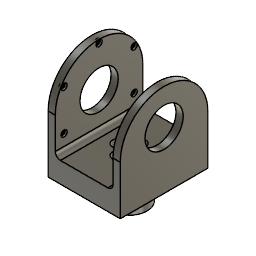
Joint 1 and 2 (Autodesk Fusion 360 archive; units mm, degrees)
design "Hinge"
Autodesk Fusion 360 part; units mm, degrees
sketch "Sketch1" plane through (0, 0, 0) normal (0, 0, 1) x (1, 0, 0)
  line L0 (0, 0) -> (70, 0)
  line L1 (70, 0) -> (70, 85)
  line L2 (70, 85) -> (0, 85)
  line L3 (0, 85) -> (0, 0)
  dimension "d1" = 70
  dimension "d2" = 85
  constraint horizontal L0
  constraint vertical L1
  constraint horizontal L2
  constraint vertical L3
  constraint coincident L0.start L3.end
  measures "d1" distance of L0.start L0.end
  measures "d2" distance of L0.start L2.end
extrude "Extrude1" add sketch "Sketch1" along normal blind 20
sketch "Sketch2" plane through (0, 0, 20) normal (0, 0, 1) x (-1, 0, 0)
  line L0 (0, -85) -> (0, 0)
  line L1 (0, 0) -> (-70, 0)
  line L2 (-70, 0) -> (-70, -85)
  line L3 (-70, -85) -> (0, -85)
  line L4 (-70, 0) -> (-63, 0)
  line L5 (-63, 0) -> (-63, -85)
  line L6 (-63, -85) -> (-70, -85)
  line L7 (-70, -85) -> (-70, 0)
  line L8 (0, 0) -> (-7, 0)
  line L9 (-7, 0) -> (-7, -85)
  line L10 (-7, -85) -> (0, -85)
  line L11 (0, -85) -> (0, 0)
  dimension "d5" = 7
  dimension "d6" = 7
  constraint horizontal L4
  constraint vertical L5
  constraint horizontal L6
  constraint vertical L7
  constraint coincident L1.end L2.start
  constraint horizontal L8
  constraint vertical L9
  constraint horizontal L10
  constraint vertical L11
  constraint coincident L0.end L1.start
  measures "d5" distance of L1.end L4.end
  measures "d6" distance of L0.end L8.end
extrude "Extrude2" add sketch "Sketch2" along normal blind 70 contours L1 L2 L3 L4 L5 L6 L7
extrude "Extrude3" add sketch "Sketch2" along normal blind 78 contours L0 L1 L3 L8 L9 L10 L11
sketch "Sketch3" plane through (0, 0, 0) normal (-1, 0, 0) x (0, -1, 0)
  line L0 (-85, 0) -> (0, 0)
  line L1 (0, 0) -> (0, 98)
  line L2 (0, 98) -> (-85, 98)
  line L3 (-85, 98) -> (-85, 0)
  circle A0 centre (-42.5, 55.5) radius 18.5
  dimension "d11" = 37
  dimension "d12" = 42.5
  dimension "d13" = 42.5
  measures "d11" diameter of A0
  measures "d12" distance of L2 A0.centre
  measures "d13" distance of L3 A0.centre
extrude "Extrude4" cut sketch "Sketch3" against normal blind 70 contours A0
fillet "Fillet1" radius 42.5 2 edges at (3.5, 0, 98) (3.5, 85, 98)
fillet "Fillet2" radius 42.5 2 edges at (66.5, 0, 90) (66.5, 85, 90)
fillet "Fillet3" radius 5 2 edges at (63, 42.5, 20) (7, 42.5, 20)
sketch "Sketch4" plane through (0, 0, 0) normal (-1, 0, 0) x (0, -1, 0)
  arc A0 (0, 55.5) -> (-85, 55.5) centre (-42.5, 55.5) ccw
  line L0 (-85, 55.5) -> (-85, 0)
  line L1 (-85, 0) -> (0, 0)
  line L2 (0, 0) -> (0, 55.5)
  circle A1 centre (-42.5, 55.5) radius 18.5
  circle A2 centre (-42.5, 55.5) radius 39.25
  circle A3 centre (-42.5, 94.75) radius 1.65
  circle A4 centre (-8.5085, 75.125) radius 1.65
  circle A5 centre (-76.4915, 75.125) radius 1.65
  circle A6 centre (-76.4915, 35.875) radius 1.65
  circle A7 centre (-8.5085, 35.875) radius 1.65
  line L3 (-42.5, 94.75) -> (-42.5, 55.5)
  line L4 (-42.5, 55.5) -> (-8.5085, 75.125)
  dimension "d22" = 78.5
  dimension "d23" = 3.3
  dimension "d24" = 3.3
  dimension "d25" = 3.3
  dimension "d26" = 3.3
  dimension "d27" = 3.3
  dimension "d65" = 60
  constraint concentric A0 A2
  constraint coincident A2 A3.centre
  constraint coincident A2 A5.centre
  constraint coincident A2 A6.centre
  constraint coincident A2 A7.centre
  constraint coincident A3.centre L3.start
  constraint coincident A0.centre A1.centre
  constraint vertical L3
  constraint coincident A2 A4.centre
  measures "d22" diameter of A2
  measures "d23" diameter of A3
  measures "d24" diameter of A4
  measures "d25" diameter of A5
  measures "d26" diameter of A6
  measures "d27" diameter of A7
  measures "d65" angle of L3 L4
extrude "Extrude5" cut sketch "Sketch4" against normal blind 7 contours A2 A4 L4 | A2 A4 L4 | A2 A3 L3 | A2 A3 L3 | A2 A4 | A2 A3 | A2 A5 | A2 A5 | A2 A7 | A2 A7 | A2 A6 | A2 A6
sketch "Sketch5" plane through (7, 0, 0) normal (1, 0, 0) x (0, 1, 0)
  circle A0 centre (76.4915, 35.875) radius 1.65
  circle A1 centre (76.4915, 75.125) radius 1.65
  circle A2 centre (8.5085, 35.875) radius 1.65
  circle A3 centre (42.5, 94.75) radius 1.65
  circle A4 centre (8.5085, 75.125) radius 1.65
  line L0 (0, 25) -> (85, 25)
  line L1 (85, 25) -> (85, 55.5)
  arc A5 (85, 55.5) -> (0, 55.5) centre (42.5, 55.5) ccw
  line L2 (0, 55.5) -> (0, 25)
  circle A6 centre (42.5, 55.5) radius 18.5
  circle A7 centre (42.5, 94.75) radius 3
  circle A8 centre (76.4915, 75.125) radius 3
  circle A9 centre (8.5085, 75.125) radius 3
  circle A10 centre (8.5085, 35.875) radius 3
  circle A11 centre (76.4915, 35.875) radius 3
  dimension "d30" = 6
  dimension "d31" = 6
  dimension "d32" = 6
  dimension "d33" = 6
  dimension "d34" = 6
  constraint concentric A3 A7
  constraint concentric A1 A8
  constraint concentric A4 A9
  constraint concentric A2 A10
  constraint concentric A0 A11
  measures "d30" diameter of A7
  measures "d31" diameter of A8
  measures "d32" diameter of A9
  measures "d33" diameter of A10
  measures "d34" diameter of A11
extrude "Extrude6" cut sketch "Sketch5" against normal blind 2 contours A7 | A8 | A9 | A10 | A11
sketch "Sketch6" plane through (0, 0, 0) normal (0, 0, -1) x (1, 0, 0)
  line L0 (0, 0) -> (0, -85)
  line L1 (0, -85) -> (70, -85)
  line L2 (70, -85) -> (70, 0)
  line L3 (70, 0) -> (0, 0)
  circle A0 centre (36, -42.5) radius 30.5
  point P0 (58, -42.5)
  point P1 (36, -42.5)
  dimension "d37" = 42.5
  dimension "d38" = 12
  dimension "d39" = 22
  dimension "d40" = 42.5
  dimension "d41" = 61
  constraint coincident P1 A0.centre
  measures "d37" distance of L3 P0
  measures "d38" distance of L2 P0
  measures "d39" distance of P0 P1
  measures "d40" distance of L3 P1
  measures "d41" diameter of A0
extrude "Extrude7" cut sketch "Sketch6" against normal blind 10 contours A0
sketch "Sketch7" plane through (0, 0, 10) normal (0, 0, -1) x (1, 0, 0)
  circle A0 centre (36, -42.5) radius 30.5
  circle A1 centre (36, -42.5) radius 17.5
  dimension "d44" = 35
  constraint concentric A0 A1
  measures "d44" diameter of A1
extrude "Extrude8" add sketch "Sketch7" along normal blind 33 contours A1
sketch "Sketch8" plane through (0, 0, -23) normal (0, 0, -1) x (1, 0, 0)
  circle A0 centre (36, -42.5) radius 17.5
  circle A1 centre (36, -32.5) radius 2.65
  circle A2 centre (36, -52.5) radius 2.65
  circle A3 centre (46, -42.5) radius 2.65
  circle A4 centre (26, -42.5) radius 2.65
  dimension "d47" = 5.3
  dimension "d48" = 10
  dimension "d49" = 5.3
  dimension "d50" = 10
  dimension "d51" = 5.3
  dimension "d52" = 10
  dimension "d53" = 5.3
  dimension "d54" = 10
  dimension "d55" = 10
  dimension "d56" = 10
  measures "d47" diameter of A1
  measures "d48" distance of A0.centre A1.centre
  measures "d49" diameter of A2
  measures "d50" distance of A0.centre A2.centre
  measures "d51" diameter of A3
  measures "d52" distance of A0.centre A3.centre
  measures "d53" diameter of A4
  measures "d54" distance of A0.centre A4.centre
  measures "d55" vertical distance of A2.centre A3.centre
  measures "d56" vertical distance of A2.centre A4.centre
extrude "Extrude9" cut sketch "Sketch8" against normal blind 48 contours A1 | A2 | A3 | A4
sketch "Sketch9" plane through (0, 0, 20) normal (0, 0, 1) x (-1, 0, 0)
  circle A0 centre (-36, -32.5) radius 2.65
  circle A1 centre (-26, -42.5) radius 2.65
  circle A2 centre (-46, -42.5) radius 2.65
  circle A3 centre (-36, -52.5) radius 2.65
  line L0 (-12, -85) -> (-12, 0)
  line L1 (-12, 0) -> (-58, 0)
  line L2 (-58, 0) -> (-58, -85)
  line L3 (-58, -85) -> (-12, -85)
  circle A4 centre (-36, -52.5) radius 6
  circle A5 centre (-26, -42.5) radius 6
  circle A6 centre (-46, -42.5) radius 6
  circle A7 centre (-36, -32.5) radius 6
  dimension "d59" = 12
  dimension "d60" = 12
  dimension "d61" = 12
  dimension "d62" = 12
  constraint concentric A3 A4
  constraint concentric A1 A5
  constraint concentric A2 A6
  constraint concentric A0 A7
  measures "d59" diameter of A4
  measures "d60" diameter of A5
  measures "d61" diameter of A6
  measures "d62" diameter of A7
extrude "Extrude10" cut sketch "Sketch9" against normal blind 12 contours A4 | A5 | A6 | A7

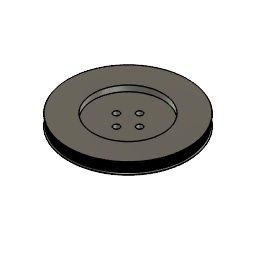
design "GT2-120"
Autodesk Fusion 360 part; units mm, degrees
sketch "Pulley Cylinder" plane through (0, 0, 0) normal (0, 0, 1) x (1, 0, 0) in component "Component"
  circle A0 centre (0, 0) radius 50.675582
extrude "Extrude1" add sketch "Pulley Cylinder" along normal blind 7 contours A0 picked at (-11.093693, -15.667951) in component "Component"
ref_plane "WorkPlane1" through (0, 0, 7) normal (0, 0, 1) x (1, 0, 0) in component "Component"
sketch "Sketch2" plane through (0, 0, 7) normal (0, 0, 1) x (1, 0, 0) in component "Component"
  circle A0 centre (0, 0) radius 51.675582
ref_plane "WorkPlane2" through (0, 0, 0) normal (0, 0, 1) x (1, 0, 0) in component "Component"
sketch "Sketch3" plane through (0, 0, 0) normal (0, 0, 1) x (1, 0, 0) in component "Component"
  circle A0 centre (0, 0) radius 51.675582
extrude "Extrude2" add sketch "Sketch2" along normal blind 1.5 contours A0 picked at (-10.126036, -19.823905) in component "Component"
extrude "Extrude3" add sketch "Sketch3" against normal blind 1.5 contours A0 picked at (-10.126036, -19.823905) in component "Component"
chamfer "Chamfer1" distance 1 angle 45 1 edges at (-48.178558, -18.686688, 0) in component "Component"
chamfer "Chamfer2" distance 1 angle 45 1 edges at (-48.178558, -18.686688, 7) in component "Component"
chamfer "Chamfer3" distance 0.2 angle 45 1 edges at (-48.178558, 18.686688, -1.5) in component "Component"
chamfer "Chamfer4" distance 0.2 angle 45 1 edges at (-48.178558, -18.686688, 8.5) in component "Component"
sketch "Bore" plane through (0, 0, 0) normal (0, 0, 1) x (1, 0, 0) in component "Component"
  circle A0 centre (0, 0) radius 1.5
  constraint coincident A0.centre origin
extrude "Extrude4" cut sketch "Bore" along normal blind 8.5 and the other way blind 1.5 contours A0 picked at (0.826239, -0.56332) in component "Component"
sketch "Tooth Profile" plane through (0, 0, 0) normal (0, 0, 1) x (1, 0, 0) in component "Component"
  circle A0 centre (0, 0) radius 50.675582 construction
  line L0 (-76.013373, 0) -> (76.013373, 0) construction
  line L1 (50.675582, -50.675582) -> (50.675582, 50.675582) construction
  line L2 (49.773989, 0.401771) -> (50.673989, 0.401771) construction
  line L3 (49.773989, -0.401771) -> (50.673989, -0.401771) construction
  arc A1 (50.097805, 0.401771) -> (50.097805, -0.401771) centre (50.48033, 0) ccw
  line L4 (49.925582, 0.4) -> (49.925582, -0.4) construction
  line L5 (50.097805, 0.401771) -> (50.097805, -0.401771) construction
  arc A2 (50.230073, -0.494298) -> (50.540254, -0.589246) centre (50.673989, 0.401771) ccw
  arc A3 (50.540254, 0.589247) -> (50.230083, 0.494303) centre (50.673989, -0.401771) ccw
  arc A4 (50.540254, 0.589247) -> (50.670177, 0.74009) centre (50.520193, 0.737899) ccw
  arc A5 (50.230083, 0.494303) -> (50.097805, 0.401771) centre (50.469126, 0.011768) ccw
  arc A6 (50.670177, -0.740089) -> (50.540254, -0.589246) centre (50.520193, -0.737899) ccw
  arc A7 (50.097805, -0.401771) -> (50.230073, -0.494298) centre (50.469115, -0.01178) ccw
  arc A8 (50.670177, -0.740089) -> (50.670177, 0.74009) centre (0, 0) ccw
  point P0 (50.48033, 0)
  point P1 (50.480582, 0)
  point P2 (50.480582, 0)
  dimension "d17" = 101.351164
  dimension "d18" = 0.803543
  dimension "d19" = 0.75
  dimension "d20" = 0.577777
  dimension "d21" = 1
  dimension "d22" = 1
  dimension "d23" = 0.15
  dimension "d24" = 0.15
  constraint coincident A0.centre A8.centre
  constraint midpoint A0.centre L0
  constraint horizontal L0
  constraint vertical L1
  constraint tangent A0 L1
  constraint horizontal L2
  constraint vertical L4
  constraint tangent A1 L4
  constraint tangent A3 A4
  constraint tangent A0 A4
  constraint tangent A1 A5
  constraint tangent A3 A5
  constraint tangent A2 A6
  constraint tangent A0 A6
  constraint tangent A1 A7
  constraint tangent A2 A7
  measures "d17" diameter of A0
  measures "d21" radius of A2
  measures "d22" radius of A3
  measures "d23" radius of A4
  measures "d24" radius of A6
extrude "Extrude5" cut sketch "Tooth Profile" along normal blind 7 contours A1 A2 A3 A4 A5 A6 A7 A8 picked at (50.425682, 0.013603) in component "Component"
pattern_circular "C-Pattern1" count 160 over 360 about axis through (0, 0, 1.75) along (0, 0, 1) of "Extrude5" in component "Component"
sketch "Sketch1" plane through (0, 0, 8.5) normal (0, 0, 1) x (-1, 0, 0)
  circle A0 centre (0, 0) radius 1.5
  circle A1 centre (0, 0) radius 51.475582
  circle A2 centre (0, 0) radius 30
  dimension "d29" = 60
  constraint coincident A0.centre A1.centre
  measures "d29" diameter of A2
extrude "Extrude6" cut sketch "Sketch1" against normal blind 5 contours A2 picked at (20.382724, -1.564944) in component "Component"
sketch "Sketch2 (2)" plane through (0, 0, 3.5) normal (0, 0, 1) x (-1, 0, 0)
  circle A0 centre (0, 0) radius 1.5
  circle A1 centre (0, 0) radius 30
  circle A2 centre (0, -10) radius 2.65
  circle A3 centre (10, 0) radius 2.65
  circle A4 centre (0, 10) radius 2.65
  circle A5 centre (-10, 0) radius 2.65
  dimension "d32" = 5.3
  dimension "d33" = 10
  dimension "d34" = 5.3
  dimension "d35" = 10
  dimension "d36" = 5.3
  dimension "d37" = 10
  dimension "d38" = 5.3
  dimension "d39" = 10
  measures "d32" diameter of A2
  measures "d33" distance of A0.centre A2.centre
  measures "d34" diameter of A3
  measures "d35" distance of A0.centre A3.centre
  measures "d36" diameter of A4
  measures "d37" distance of A0.centre A4.centre
  measures "d38" diameter of A5
  measures "d39" distance of A0.centre A5.centre
extrude "Extrude7" cut sketch "Sketch2 (2)" against normal blind 5 contours A2 | A3 | A4 | A5 picked at (0.676907, -9.00716) picked at (10.424592, 0.99284) picked at (0.921701, 9.488023) picked at (-9.581274, 0.690618) in component "Component"
delete_face "DeleteFace1" 1 faces at (1.498135, -0.074769, 1.833333) in component "Component"
sketch "Sketch3 (2)" plane through (0, 0, -1.5) normal (0, 0, -1) x (1, 0, 0)
  circle A0 centre (-10, 0) radius 2.65
  circle A1 centre (0, 10) radius 2.65
  circle A2 centre (0, -10) radius 2.65
  circle A3 centre (10, 0) radius 2.65
  circle A4 centre (0, 0) radius 51.475582
  circle A5 centre (0, 0) radius 4
  dimension "d42" = 8
  constraint coincident A4.centre A5.centre
  measures "d42" diameter of A5
extrude "Extrude8" add sketch "Sketch3 (2)" along normal blind 12 contours A5 picked at (-1.245636, 0.013218) in component "Component"
component "Component" placed x (1, 0, 0) y (0, 1, 0) z (0, 0, 1) at (0, 0, 0)
named bodies: "GT2 Pulley"

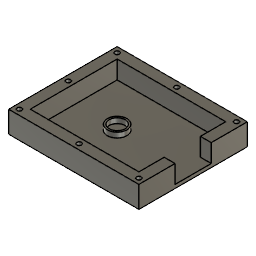
design "Box bottom"
Autodesk Fusion 360 part; units mm, degrees
sketch "Sketch1" plane through (0, 0, 0) normal (0, 0, 1) x (1, 0, 0)
  line L0 (0, 0) -> (180, 0)
  line L1 (180, 0) -> (180, 150)
  line L2 (180, 150) -> (0, 150)
  line L3 (0, 150) -> (0, 0)
  dimension "d1" = 180
  dimension "d2" = 150
  constraint horizontal L0
  constraint vertical L1
  constraint horizontal L2
  constraint vertical L3
  constraint coincident L0.start L3.end
  measures "d1" distance of L0.start L0.end
  measures "d2" distance of L0.start L2.end
extrude "Extrude1" add sketch "Sketch1" along normal blind 5
sketch "Sketch2" plane through (0, 0, 5) normal (0, 0, 1) x (-1, 0, 0)
  line L0 (0, -150) -> (0, 0)
  line L1 (0, 0) -> (-180, 0)
  line L2 (-180, 0) -> (-180, -150)
  line L3 (-180, -150) -> (0, -150)
  circle A0 centre (-75, -75) radius 11
  circle A1 centre (-75, -75) radius 13.5
  dimension "d5" = 22
  dimension "d6" = 75
  dimension "d7" = 75
  dimension "d8" = 27
  constraint concentric A0 A1
  measures "d5" diameter of A0
  measures "d6" distance of L3 A0.centre
  measures "d7" distance of L0 A0.centre
  measures "d8" diameter of A1
extrude "Extrude2" add sketch "Sketch2" along normal blind 7 contours A1
sketch "Sketch3" plane through (0, 0, 5) normal (0, 0, 1) x (-1, 0, 0)
  line L0 (0, -150) -> (0, 0)
  line L1 (0, 0) -> (-180, 0)
  line L2 (-180, 0) -> (-180, -150)
  line L3 (-180, -150) -> (0, -150)
  circle A0 centre (-75, -75) radius 13.5
  line L4 (-15, -15) -> (-165, -15)
  line L5 (-165, -135) -> (-15, -135)
  line L6 (-15, -135) -> (-15, -15)
  line L7 (-165, -50) -> (-180, -50)
  line L8 (-165, -100) -> (-180, -100)
  line L9 (-165, -135) -> (-165, -100)
  line L10 (-165, -15) -> (-165, -50)
  dimension "d11" = 150
  dimension "d12" = 120
  dimension "d13" = 15
  dimension "d14" = 15
  dimension "d17" = 25
  dimension "d18" = 25
  constraint horizontal L4
  constraint horizontal L5
  constraint vertical L6
  constraint coincident L2 L7.end
  constraint perpendicular L2 L7
  constraint coincident L2 L8.end
  constraint perpendicular L2 L8
  constraint perpendicular L8 L9
  constraint perpendicular L7 L10
  measures "d11" distance of L4.start L4.end
  measures "d12" distance of L4.start L5.end
  measures "d13" distance of L0 L6
  measures "d14" distance of L1 L4
  measures "d17" distance of A0.centre L7
  measures "d18" distance of A0.centre L8
extrude "Extrude4" add sketch "Sketch3" along normal blind 25 contours L0 L1 L2 L3 L4 L5 L6 L7 L8 L9 L10
sketch "Sketch4" plane through (0, 0, 30) normal (0, 0, 1) x (-1, 0, 0)
  line L0 (-165, -135) -> (-165, -100)
  line L1 (-165, -100) -> (-180, -100)
  line L2 (-180, -100) -> (-180, -150)
  line L3 (-180, -150) -> (0, -150)
  line L4 (0, -150) -> (0, 0)
  line L5 (0, 0) -> (-180, 0)
  line L6 (-180, 0) -> (-180, -50)
  line L7 (-180, -50) -> (-165, -50)
  line L8 (-165, -50) -> (-165, -15)
  line L9 (-165, -15) -> (-15, -15)
  line L10 (-15, -15) -> (-15, -135)
  line L11 (-15, -135) -> (-165, -135)
  circle A0 centre (-7.5, -142.5) radius 3.2
  circle A1 centre (-7.5, -75) radius 3.2
  circle A2 centre (-7.5, -7.5) radius 3.2
  circle A3 centre (-172.5, -7.5) radius 3.2
  circle A4 centre (-172.5, -142.5) radius 3.2
  circle A5 centre (-90, -142.5) radius 3.2
  circle A6 centre (-90, -7.5) radius 3.2
  dimension "d21" = 6.4
  dimension "d22" = 7.5
  dimension "d23" = 7.5
  dimension "d24" = 6.4
  dimension "d25" = 7.5
  dimension "d26" = 6.4
  dimension "d27" = 7.5
  dimension "d28" = 7.5
  dimension "d29" = 6.4
  dimension "d30" = 7.5
  dimension "d31" = 7.5
  dimension "d32" = 6.4
  dimension "d33" = 7.5
  dimension "d34" = 7.5
  dimension "d35" = 6.4
  dimension "d36" = 7.5
  dimension "d37" = 90
  dimension "d38" = 6.4
  dimension "d39" = 7.5
  dimension "d40" = 90
  measures "d21" diameter of A0
  measures "d22" distance of L3 A0.centre
  measures "d23" distance of L4 A0.centre
  measures "d24" diameter of A1
  measures "d25" distance of L4 A1.centre
  measures "d26" diameter of A2
  measures "d27" distance of L4 A2.centre
  measures "d28" distance of L5 A2.centre
  measures "d29" diameter of A3
  measures "d30" distance of L6 A3.centre
  measures "d31" distance of L5 A3.centre
  measures "d32" diameter of A4
  measures "d33" distance of L2 A4.centre
  measures "d34" distance of L3 A4.centre
  measures "d35" diameter of A5
  measures "d36" distance of L3 A5.centre
  measures "d37" distance of L2 A5.centre
  measures "d38" diameter of A6
  measures "d39" distance of L5 A6.centre
  measures "d40" distance of L6 A6.centre
extrude "Extrude5" cut sketch "Sketch4" against normal blind 10.5 contours A0 | A1 | A2 | A3 | A4 | A5 | A6

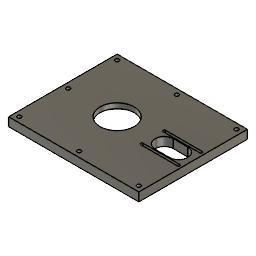
design "Box top"
Autodesk Fusion 360 part; units mm, degrees
sketch "Sketch1" plane through (0, 0, 0) normal (0, 0, 1) x (1, 0, 0)
  line L0 (0, 0) -> (180, 0)
  line L1 (180, 0) -> (180, 150)
  line L2 (180, 150) -> (0, 150)
  line L3 (0, 150) -> (0, 0)
  dimension "d1" = 180
  dimension "d2" = 150
  constraint horizontal L0
  constraint vertical L1
  constraint horizontal L2
  constraint vertical L3
  constraint coincident L0.start L3.end
  measures "d1" distance of L0.start L0.end
  measures "d2" distance of L0.start L2.end
extrude "Extrude1" add sketch "Sketch1" along normal blind 12
sketch "Sketch3" plane through (0, 0, 0) normal (0, 0, -1) x (1, 0, 0)
  line L0 (0, 0) -> (0, -150)
  line L1 (0, -150) -> (180, -150)
  line L2 (180, -150) -> (180, 0)
  line L3 (180, 0) -> (0, 0)
  circle A0 centre (75, -75) radius 30
  dimension "d8" = 60
  measures "d8" diameter of A0
extrude "Extrude3" cut sketch "Sketch3" against normal blind 5 contours A0
sketch "Sketch5" plane through (0, 0, 5) normal (0, 0, -1) x (1, 0, 0)
  circle A0 centre (75, -75) radius 30
  circle A1 centre (75, -75) radius 23.5
  dimension "d14" = 47
  constraint concentric A0 A1
  measures "d14" diameter of A1
extrude "Extrude5" cut sketch "Sketch5" against normal blind 12 contours A1
sketch "Sketch6" plane through (0, 0, 0) normal (0, 0, -1) x (1, 0, 0)
  circle A0 centre (75, -75) radius 30
  line L0 (0, 0) -> (0, -150)
  line L1 (0, -150) -> (180, -150)
  line L2 (180, -150) -> (180, 0)
  line L3 (180, 0) -> (0, 0)
  line L4 (140, -87.5) -> (160, -87.5)
  line L5 (160, -62.5) -> (140, -62.5)
  arc A1 (140, -62.5) -> (140, -87.5) centre (140, -75) ccw
  arc A2 (160, -87.5) -> (160, -62.5) centre (160, -75) ccw
  line L6 (175.5, -61.15) -> (124.5, -61.15)
  line L7 (124.5, -57.85) -> (175.5, -57.85)
  arc A3 (124.5, -57.85) -> (124.5, -61.15) centre (124.5, -59.5) ccw
  arc A4 (175.5, -61.15) -> (175.5, -57.85) centre (175.5, -59.5) ccw
  line L8 (175.5, -88.85) -> (124.5, -88.85)
  line L9 (124.5, -92.15) -> (175.5, -92.15)
  arc A5 (124.5, -88.85) -> (124.5, -92.15) centre (124.5, -90.5) ccw
  arc A6 (175.5, -92.15) -> (175.5, -88.85) centre (175.5, -90.5) ccw
  dimension "d17" = 25
  dimension "d18" = 20
  dimension "d19" = 20
  dimension "d20" = 51
  dimension "d22" = 15.5
  dimension "d23" = 3.3
  dimension "d24" = 51
  dimension "d25" = 3.3
  dimension "d29" = 15.5
  dimension "d30" = 15.5
  dimension "d31" = 75
  constraint horizontal L4
  constraint parallel L3 L5
  constraint tangent L5 A1
  constraint tangent L4 A1
  constraint tangent L5 A2
  constraint tangent L4 A2
  constraint horizontal L6
  constraint perpendicular L2 L7
  constraint tangent L7 A3
  constraint tangent L6 A3
  constraint tangent L7 A4
  constraint tangent L6 A4
  constraint parallel L6 L8
  constraint parallel L8 L9
  constraint tangent L8 A5
  constraint tangent L9 A5
  constraint tangent L8 A6
  constraint tangent L9 A6
  measures "d17" distance of L4 L5
  measures "d18" distance of A1.centre A2.centre
  measures "d19" distance of L2 A2.centre
  measures "d20" distance of L6.start L6.end
  measures "d22" horizontal distance of A1.centre L6.end
  measures "d23" distance of L6 L7
  measures "d24" distance of L8.start L8.end
  measures "d25" distance of L8 L9
  measures "d29" vertical distance of A1.centre A3.centre
  measures "d30" vertical distance of A1.centre A5.centre
  measures "d31" distance of L3 A2.centre
extrude "Extrude6" cut sketch "Sketch6" against normal blind 12 contours L4 L5 A1 A2 | L6 L7 A3 A4 | L8 L9 A5 A6
sketch "Sketch7" plane through (0, 0, 12) normal (0, 0, 1) x (-1, 0, 0)
  line L0 (-124.5, -61.15) -> (-175.5, -61.15)
  arc A0 (-175.5, -57.85) -> (-175.5, -61.15) centre (-175.5, -59.5) ccw
  line L1 (-175.5, -57.85) -> (-124.5, -57.85)
  arc A1 (-124.5, -61.15) -> (-124.5, -57.85) centre (-124.5, -59.5) ccw
  line L2 (-160, -62.5) -> (-140, -62.5)
  arc A2 (-140, -87.5) -> (-140, -62.5) centre (-140, -75) ccw
  line L3 (-140, -87.5) -> (-160, -87.5)
  arc A3 (-160, -62.5) -> (-160, -87.5) centre (-160, -75) ccw
  line L4 (-175.5, -88.85) -> (-124.5, -88.85)
  arc A4 (-124.5, -92.15) -> (-124.5, -88.85) centre (-124.5, -90.5) ccw
  line L5 (-124.5, -92.15) -> (-175.5, -92.15)
  arc A5 (-175.5, -88.85) -> (-175.5, -92.15) centre (-175.5, -90.5) ccw
  circle A6 centre (-75, -75) radius 23.5
  line L6 (0, -150) -> (0, 0)
  line L7 (0, 0) -> (-180, 0)
  line L8 (-180, 0) -> (-180, -150)
  line L9 (-180, -150) -> (0, -150)
  circle A7 centre (-7.5, -7.5) radius 2.65
  circle A8 centre (-7.5, -142.5) radius 2.65
  circle A9 centre (-172.5, -142.5) radius 2.65
  circle A10 centre (-172.5, -7.5) radius 2.65
  circle A11 centre (-90, -7.5) radius 2.65
  circle A12 centre (-90, -142.5) radius 2.65
  circle A13 centre (-7.5, -75) radius 2.65
  dimension "d32" = 5.3
  dimension "d33" = 7.5
  dimension "d34" = 7.5
  dimension "d35" = 5.3
  dimension "d36" = 7.5
  dimension "d37" = 7.5
  dimension "d38" = 5.3
  dimension "d39" = 7.5
  dimension "d40" = 7.5
  dimension "d41" = 5.3
  dimension "d42" = 7.5
  dimension "d43" = 7.5
  dimension "d44" = 5.3
  dimension "d45" = 90
  dimension "d46" = 7.5
  dimension "d47" = 5.3
  dimension "d48" = 7.5
  dimension "d49" = 90
  dimension "d50" = 5.3
  dimension "d51" = 7.5
  measures "d32" diameter of A7
  measures "d33" distance of L6 A7.centre
  measures "d34" distance of L7 A7.centre
  measures "d35" diameter of A8
  measures "d36" distance of L9 A8.centre
  measures "d37" distance of L6 A8.centre
  measures "d38" diameter of A9
  measures "d39" distance of L9 A9.centre
  measures "d40" distance of L8 A9.centre
  measures "d41" diameter of A10
  measures "d42" distance of L8 A10.centre
  measures "d43" distance of L7 A10.centre
  measures "d44" diameter of A11
  measures "d45" distance of L6 A11.centre
  measures "d46" distance of L7 A11.centre
  measures "d47" diameter of A12
  measures "d48" distance of L9 A12.centre
  measures "d49" distance of L8 A12.centre
  measures "d50" diameter of A13
  measures "d51" distance of L6 A13.centre
extrude "Extrude7" cut sketch "Sketch7" against normal blind 12 contours A7 | A8 | A9 | A10 | A11 | A12 | A13

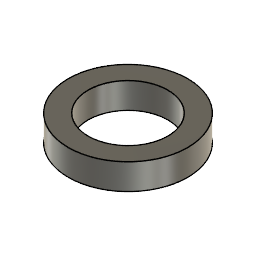
design "Thrust bearing 40x60x13"
Autodesk Fusion 360 part; units mm, degrees
sketch "Sketch1" plane through (0, 0, 0) normal (0, 0, 1) x (1, 0, 0)
  circle A0 centre (0, 0) radius 30
  circle A1 centre (0, 0) radius 20
  dimension "d1" = 60
  dimension "d2" = 40
  constraint coincident A0.centre A1.centre
  measures "d1" diameter of A0
  measures "d2" diameter of A1
extrude "Extrude1" add sketch "Sketch1" along normal blind 13

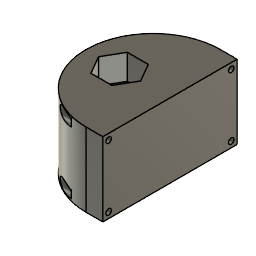
design "Coupling shaft"
Autodesk Fusion 360 part; units mm, degrees
sketch "Sketch1" plane through (0, 0, 0) normal (1, 0, 0) x (0, 1, 0)
  line L0 (0, 0) -> (-80, 0)
  line L1 (-80, 0) -> (-80, 44)
  line L2 (-80, 44) -> (0, 44)
  line L3 (0, 44) -> (0, 0)
  dimension "d1" = 80
  dimension "d2" = 44
  constraint horizontal L0
  constraint vertical L1
  constraint horizontal L2
  constraint vertical L3
  constraint coincident L0.start L3.end
  measures "d1" distance of L0.start L0.end
  measures "d2" distance of L0.start L2.end
extrude "Extrude1" add sketch "Sketch1" along normal blind 50
sketch "Sketch3" plane through (0, 0, 0) normal (-1, 0, 0) x (0, -1, 0)
  line L0 (80, 44) -> (0, 44)
  line L1 (0, 44) -> (0, 0)
  line L2 (0, 0) -> (80, 0)
  line L3 (80, 0) -> (80, 44)
  circle A0 centre (3.5, 40.5) radius 1.65
  circle A1 centre (3.5, 3.5) radius 1.65
  circle A2 centre (76.5, 40.5) radius 1.65
  circle A3 centre (76.5, 3.5) radius 1.65
  dimension "d17" = 3.3
  dimension "d18" = 3.5
  dimension "d19" = 3.5
  dimension "d20" = 3.3
  dimension "d21" = 3.5
  dimension "d22" = 3.3
  dimension "d23" = 3.5
  dimension "d24" = 3.3
  measures "d17" diameter of A0
  measures "d18" distance of L0 A0.centre
  measures "d19" distance of L1 A0.centre
  measures "d20" diameter of A1
  measures "d21" distance of L2 A1.centre
  measures "d22" diameter of A2
  measures "d23" distance of L3 A2.centre
  measures "d24" diameter of A3
extrude "Extrude3" cut sketch "Sketch3" against normal blind 50 contours A0 | A1 | A2 | A3
sketch "Sketch6" plane through (0, 0, 0) normal (-1, 0, 0) x (0, -1, 0)
  circle A0 centre (76.5, 40.5) radius 1.65
  circle A1 centre (76.5, 3.5) radius 1.65
  circle A2 centre (3.5, 40.5) radius 1.65
  circle A3 centre (3.5, 3.5) radius 1.65
  line L0 (80, 44) -> (0, 44)
  line L1 (0, 44) -> (0, 0)
  line L2 (0, 0) -> (80, 0)
  line L3 (80, 0) -> (80, 44)
  circle A4 centre (3.5, 40.5) radius 3
  circle A5 centre (3.5, 3.5) radius 3
  circle A6 centre (76.5, 40.5) radius 3
  circle A7 centre (76.5, 3.5) radius 3
  dimension "d46" = 6
  dimension "d47" = 6
  dimension "d48" = 6
  dimension "d49" = 6
  constraint concentric A2 A4
  constraint concentric A3 A5
  constraint concentric A0 A6
  constraint concentric A1 A7
  measures "d46" diameter of A4
  measures "d47" diameter of A5
  measures "d48" diameter of A6
  measures "d49" diameter of A7
extrude "Extrude7" cut sketch "Sketch6" against normal blind 30 contours A4 | A5 | A6 | A7
sketch "Sketch7" plane through (0, 0, 0) normal (0, 0, -1) x (1, 0, 0)
  line L0 (0, 80) -> (0, 0)
  line L1 (0, 0) -> (50, 0)
  line L2 (50, 0) -> (50, 80)
  line L3 (50, 80) -> (0, 80)
  circle A0 centre (20, 40) radius 16.5
  dimension "d52" = 33
  dimension "d53" = 20
  measures "d52" diameter of A0
  measures "d53" distance of L0 A0.centre
extrude "Extrude8" add sketch "Sketch7" along normal blind 3 contours A0
sketch "Sketch8" plane through (0, 0, -3) normal (0, 0, -1) x (1, 0, 0)
  circle A0 centre (20, 40) radius 16.5
  circle A1 centre (20, 40) radius 14.5
  dimension "d56" = 29
  constraint concentric A0 A1
  measures "d56" diameter of A1
extrude "Extrude9" add sketch "Sketch8" along normal blind 2 contours A1
fillet "Fillet1" radius 14 1 edges at (4.6166, -34.0333, -3)
sketch "Sketch9" plane through (0, 0, -5) normal (0, 0, -1) x (1, 0, 0)
  circle A0 centre (20, 40) radius 14.5
  circle A1 centre (20, 40) radius 12.5
  dimension "d61" = 25
  constraint concentric A0 A1
  measures "d61" diameter of A1
extrude "Extrude10" add sketch "Sketch9" along normal blind 7 contours A1
sketch "Sketch10" plane through (0, 0, 44) normal (0, 0, 1) x (-1, 0, 0)
  line L0 (0, 0) -> (0, 80)
  line L1 (0, 80) -> (-50, 80)
  line L2 (-50, 80) -> (-50, 0)
  line L3 (-50, 0) -> (0, 0)
  line L4 (-7.5, 40) -> (-13.75, 50.8253)
  line L5 (-13.75, 50.8253) -> (-26.25, 50.8253)
  line L6 (-26.25, 50.8253) -> (-32.5, 40)
  line L7 (-32.5, 40) -> (-26.25, 29.1747)
  line L8 (-26.25, 29.1747) -> (-13.75, 29.1747)
  line L9 (-13.75, 29.1747) -> (-7.5, 40)
  point P0 (-20, 40)
  dimension "d64" = 12.5
  dimension "d65" = 20
  measures "d64" distance of L4.start P0
  measures "d65" distance of L0 P0
extrude "Extrude11" cut sketch "Sketch10" against normal blind 15 contours L4 L5 L6 L7 L8 L9
fillet "Fillet2" radius 40 1 edges at (0, -80, 22)
fillet "Fillet3" radius 40 1 edges at (0, 0, 22)
